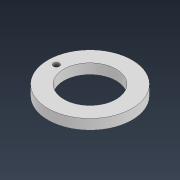
# Autodesk Inventor part: CH_02_0001_drilling_help
Saved by Autodesk Inventor 2022.3 (Build 263350030, 350C)
## iProperties
Created: 2022-08-31
Part Number: CH_02_0001_drilling_help
Material: Generic
Document SubType Name: Modeling
Designer: Tomasz Krakowski
Density: 1 g/cm^3
Appearance: Default
Author: Tomasz Krakowski
Autodesk Inventor part; units mm, degrees
ref_plane "YZ Plane" through (0, 0, 0) normal (1, 0, 0) x (0, 1, 0)
ref_plane "XZ Plane" through (0, 0, 0) normal (0, 1, 0) x (-1, 0, 0)
ref_plane "XY Plane" through (0, 0, 0) normal (0, 0, 1) x (1, 0, 0)
sketch "Sketch1" plane through (0, 0, 0) normal (0, 1, 0) x (-1, 0, 0)
  circle A0 centre (0, 0) radius 15.55
  circle A1 centre (0, 0) radius 25
  circle A2 centre (0, 0) radius 20 construction
  circle A3 centre (20, 0) radius 1.75
  line L0 (20, 0) -> (0, 0) construction
  dimension "d1" = 40
  dimension "d0" = 31.1
  dimension "d2" = 3.5
  dimension "d3" = 50
  constraints: 3 centre point, 3 coincident, 2 end point, 1 horizontal, 1 horizontal alignment, 2 other
  measures "d0" diameter of A0
  measures "d2" diameter of A3
  measures "d3" diameter of A1
extrude "Extrusion1" add sketch "Sketch1" along normal blind 6
body "Solid1"
